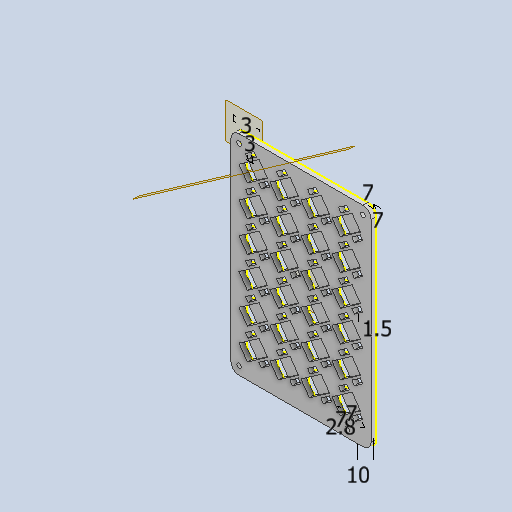
# Autodesk Inventor part: Omniscope_mid_level_v0
Saved by Autodesk Inventor 2022 (Build 260153000, 153)
## iProperties
Created: 2022-05-25
Part Number: Omniscope_mid_level_v0
Material: Generisch
Document SubType Name: Modeling
Designer: diederichbenedict
Density: 1 g/cm^3
Appearance: Vorgabe
Author: diederichbenedict
Autodesk Inventor part; units mm, degrees
ref_plane "YZ Plane" through (0, 0, 0) normal (1, 0, 0) x (0, 1, 0)
ref_plane "XZ Plane" through (0, 0, 0) normal (0, 1, 0) x (-1, 0, 0)
ref_plane "Arbeitsebene4" through (0, 0, 0) normal (0, 0, 1) x (1, 0, 0)
sketch "Skizze1" plane through (0, 0, 0) normal (0, 0, 1) x (1, 0, 0)
  circle A0 centre (37.75, -58.75) radius 1.4 projected
  circle A1 centre (37.75, 58.75) radius 1.4 projected
  circle A2 centre (-37.75, 58.75) radius 1.4 projected
  circle A3 centre (-37.75, -58.75) radius 1.4 projected
  circle A4 centre (-28.35, -47.25) radius 8 projected
  circle A5 centre (-28.35, -28.35) radius 8 projected
  circle A6 centre (-28.35, -9.45) radius 8 projected
  circle A7 centre (-28.35, 9.45) radius 8 projected
  circle A8 centre (-28.35, 28.35) radius 8 projected
  circle A9 centre (-28.35, 47.25) radius 8 projected
  circle A10 centre (-9.45, -47.25) radius 8 projected
  circle A11 centre (-9.45, -28.35) radius 8 projected
  circle A12 centre (-9.45, -9.45) radius 8 projected
  circle A13 centre (-9.45, 9.45) radius 8 projected
  circle A14 centre (-9.45, 28.35) radius 8 projected
  circle A15 centre (-9.45, 47.25) radius 8 projected
  circle A16 centre (9.45, -47.25) radius 8 projected
  circle A17 centre (9.45, -28.35) radius 8 projected
  circle A18 centre (9.45, -9.45) radius 8 projected
  circle A19 centre (9.45, 9.45) radius 8 projected
  circle A20 centre (9.45, 28.35) radius 8 projected
  circle A21 centre (9.45, 47.25) radius 8 projected
  circle A22 centre (28.35, -47.25) radius 8 projected
  circle A23 centre (28.35, -28.35) radius 8 projected
  circle A24 centre (28.35, -9.45) radius 8 projected
  circle A25 centre (28.35, 9.45) radius 8 projected
  circle A26 centre (28.35, 28.35) radius 8 projected
  arc A27 (37.75, -63.75) -> (42.75, -58.75) centre (37.75, -58.75) ccw projected
  line L0 (42.75, -58.75) -> (42.75, 58.75) projected
  arc A28 (42.75, 58.75) -> (37.75, 63.75) centre (37.75, 58.75) ccw projected
  line L1 (37.75, 63.75) -> (-37.75, 63.75) projected
  arc A29 (-37.75, 63.75) -> (-42.75, 58.75) centre (-37.75, 58.75) ccw projected
  line L2 (-42.75, 58.75) -> (-42.75, -58.75) projected
  arc A30 (-42.75, -58.75) -> (-37.75, -63.75) centre (-37.75, -58.75) ccw projected
  line L3 (-37.75, -63.75) -> (37.75, -63.75) projected
  circle A31 centre (28.35, 47.25) radius 8 projected
  line L4 (41.25, 58.75) -> (41.25, -58.75)
  arc A32 (37.75, -62.25) -> (41.25, -58.75) centre (37.75, -58.75) ccw
  line L5 (37.75, -62.25) -> (-37.75, -62.25)
  arc A33 (-41.25, -58.75) -> (-37.75, -62.25) centre (-37.75, -58.75) ccw
  line L6 (-41.25, -58.75) -> (-41.25, 58.75)
  arc A34 (-37.75, 62.25) -> (-41.25, 58.75) centre (-37.75, 58.75) ccw
  line L7 (-37.75, 62.25) -> (37.75, 62.25)
  arc A35 (41.25, 58.75) -> (37.75, 62.25) centre (37.75, 58.75) ccw
  line L8 (-34.75, 62.25) -> (-34.75, 55.75)
  line L9 (-34.75, 55.75) -> (-41.25, 55.75)
  line L10 (-32.5541, -62.25) -> (-32.5541, -54.8048)
  line L11 (-32.5541, -54.8048) -> (-41.25, -54.8048)
  line L12 (41.25, 55.25) -> (34.25, 55.25)
  line L13 (34.25, 55.25) -> (34.25, 62.25)
  line L14 (31.25, -62.25) -> (24.25, -62.25)
  line L15 (24.25, -62.25) -> (24.25, -55.25)
  line L16 (24.25, -55.25) -> (31.25, -55.25)
  line L17 (31.25, -55.25) -> (31.25, -62.25)
  circle A36 centre (28.25, -59.25) radius 1.4
  point P0 (0, 0)
  point P1 (24.25, -62.25)
  dimension "d0" = 1.5
  dimension "d1" = 3
  dimension "d2" = 3
  dimension "d5" = 7
  dimension "d6" = 7
  dimension "d7" = 7
  dimension "d8" = 7
  dimension "d9" = 10
  dimension "d10" = 2.8
  constraints: 28 end point, 8 point on circle, 7 point on line, 5 centre point, 4 perpendicular, 2 horizontal, 2 parallel, 2 vertical, 7 other
  measures "d0" distance between parallel lines of L0 L4
  measures "d1" distance from line of A2.centre L8
  measures "d2" distance from line of A2.centre L9
  measures "d5" distance between parallel lines of L13 L4
  measures "d6" distance between parallel lines of L7 L12
  measures "d7" distance of L15.end L16.end
  measures "d8" distance of L14.end L15.end
  measures "d9" distance between parallel lines of L17 L4
  measures "d10" diameter of A36
ref_plane "Arbeitsebene2" through (23.1342, 37.0359, 54) normal (0, 0, 1) x (0.8192, 0.5736, 0)
ref_plane "Arbeitsebene6" through (-37.75, 63.75, 0) normal (0, 0, 1) x (1, 0, 0)
sketch "Skizze2" plane through (-37.75, 63.75, 0) normal (0, 0, 1) x (1, 0, 0)
  circle A0 centre (66, -123) radius 1.4 projected
  circle A1 centre (75.5, -5) radius 1.4 projected
  line L0 (72, -1.5) -> (3, -1.5) projected
  line L1 (72, -8.5) -> (72, -1.5) projected
  line L2 (79, -8.5) -> (72, -8.5) projected
  line L3 (79, -122.5) -> (79, -8.5) projected
  arc A2 (75.5, -126) -> (79, -122.5) centre (75.5, -122.5) ccw projected
  line L4 (69, -126) -> (75.5, -126) projected
  line L5 (69, -119) -> (69, -126) projected
  line L6 (62, -119) -> (69, -119) projected
  line L7 (62, -126) -> (62, -119) projected
  line L8 (5.1959, -126) -> (62, -126) projected
  line L9 (5.1959, -118.5548) -> (5.1959, -126) projected
  line L10 (-3.5, -118.5548) -> (5.1959, -118.5548) projected
  line L11 (-3.5, -8) -> (-3.5, -118.5548) projected
  line L12 (3, -8) -> (-3.5, -8) projected
  line L13 (3, -1.5) -> (3, -8) projected
  circle A3 centre (0, -122.5) radius 1.4 projected
  circle A4 centre (0, -5) radius 1.4 projected
  arc A5 (75.5, -127.5) -> (80.5, -122.5) centre (75.5, -122.5) ccw projected
  line L14 (80.5, -5) -> (80.5, -122.5) projected
  arc A6 (80.5, -5) -> (75.5, 0) centre (75.5, -5) ccw projected
  line L15 (0, 0) -> (75.5, 0) projected
  arc A7 (0, 0) -> (-5, -5) centre (0, -5) ccw projected
  line L16 (-5, -122.5) -> (-5, -5) projected
  arc A8 (-5, -122.5) -> (0, -127.5) centre (0, -122.5) ccw projected
  line L17 (75.5, -127.5) -> (0, -127.5) projected
  point P0 (37.75, -63.75)
extrude "Extrusion2" add sketch "Skizze2" along normal blind 3 contours L1 L2 L3 A2 L4 L5 L6 L7 L8 L9 L10 L11 L12 L13 L0 | L17 A8 L16 A7 L15 A6 L14 A5
sketch "Skizze3" plane through (-37.75, 63.75, 3) normal (0, 0, 1) x (1, 0, 0)
  line L0 (5.0851, -23.4415) -> (-0.0771, -16.0691)
  line L1 (1.5612, -14.9219) -> (6.7234, -22.2943)
  line L2 (6.7234, -22.2943) -> (5.0851, -23.4415)
  line L3 (5.0851, -23.4415) -> (-1.8803, -10.007) construction
  line L4 (13.3163, -26.6806) -> (28.3163, -26.6806) construction
  line L5 (6.7234, -22.2943) -> (1.5612, -14.9219)
  line L6 (1.5612, -14.9219) -> (4.8378, -12.6276)
  line L7 (4.8378, -12.6276) -> (10, -20)
  line L8 (10, -20) -> (6.7234, -22.2943)
  line L9 (1.5612, -14.9219) -> (-0.0771, -16.0691)
  point P0 (37.75, -63.75)
  point P1 (1.6024, -16.7242)
  dimension "d15" = 125
  dimension "d19" = 9
  dimension "d20" = 6
  constraints: 20 end point, 3 parallel, 2 perpendicular, 1 horizontal, 1 midpoint
  measures "d15" angle of L4 L0
  measures "d19" distance between parallel lines of L6 L8
  measures "d20" distance between parallel lines of L0 L7
extrude "Extrusion3" cut sketch "Skizze3" against normal blind 55
sketch "Skizze4" plane through (-37.75, 63.75, 3) normal (0, 0, 1) x (1, 0, 0)
  line L0 (4.8378, -12.6276) -> (10, -20) projected
  line L1 (5.0851, -23.4415) -> (10, -20) projected
  line L2 (10, -20) -> (4.8378, -12.6276)
  line L3 (4.8378, -12.6276) -> (12.2102, -7.4654)
  line L4 (12.2102, -7.4654) -> (17.3724, -14.8378)
  line L5 (17.3724, -14.8378) -> (10, -20)
  point P0 (37.75, -63.75)
  dimension "d35" = 9
  constraints: 8 end point, 2 parallel, 2 perpendicular
  measures "d35" distance of L0.start L3.end
extrude "Extrusion4" cut sketch "Skizze4" against normal blind 1
sketch "Skizze5" plane through (-37.75, 63.75, 3) normal (0, 0, 1) x (1, 0, 0)
  line L0 (17.934, -18.1679) -> (13.3468, -21.3799) projected
  line L1 (17.0736, -16.9392) -> (12.4864, -20.1512) projected
  line L2 (16.5001, -16.12) -> (11.9128, -19.3321) projected
  line L3 (17.0736, -16.9392) -> (12.4864, -20.1512) projected
  line L4 (38.9474, -3.3011) -> (0.1922, -30.4378)
  line L5 (12.0686, -20.0775) -> (17.1473, -16.5214)
  line L6 (17.1473, -16.5214) -> (18.696, -18.7331)
  line L7 (18.696, -18.7331) -> (13.6172, -22.2892)
  line L8 (13.6172, -22.2892) -> (12.0686, -20.0775)
  line L9 (12.0686, -20.0775) -> (18.696, -18.7331) construction
  line L10 (17.1473, -16.5214) -> (13.6172, -22.2892) construction
  line L11 (16.5001, -16.12) -> (17.0736, -16.9392) projected
  line L12 (12.4864, -20.1512) -> (11.9128, -19.3321) projected
  point P0 (37.75, -63.75)
  point P1 (15.3823, -19.4053)
  dimension "d40" = 2.5
  dimension "d41" = 2.7
  dimension "d42" = 0.3
  dimension "d51" = 0.3
  dimension "d52" = 0.3
  constraints: 14 end point, 3 parallel, 2 midpoint, 1 perpendicular, 3 other
  measures "d40" distance between parallel lines of L0 L2
  measures "d41" distance between parallel lines of L7 L5
  measures "d42" distance between parallel lines of L5 L1
  measures "d51" distance from line of L8 L0.end
  measures "d52" distance from line of L0.start L6
extrude "Extrusion5" cut sketch "Skizze5" against normal through all contours L11 L5 L6 L4 L8 L12 L1 | L1 L12 L5 L11 | L6 L7 L8 L4
ref_plane "Arbeitsebene7" through (-35.246, 43.9947, 3) normal (-0.5736, 0.8192, 0) x (0.8192, 0.5736, 0)
mirror "Spiegeln1" about plane through (-35.246, 43.9947, 3) normal (-0.5736, 0.8192, 0) of "Extrusion5"
pattern_linear "Rechteckige Anordnung3" count 6 spacing 18.9 along (0, -1, 0) count 4 spacing 18.9 along (1, 0, 0) of "Extrusion3", "Extrusion4", "Extrusion5", "Spiegeln1"
